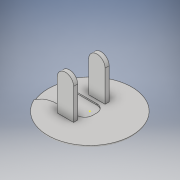
# Autodesk Inventor part: Replacemnet part(wall socket)
Saved by Autodesk Inventor 2018 (Build 220112000, 112)
## iProperties
Created: 2019-02-07
Part Number: Replacemnet part(wall socket)
Material: Generic
Document SubType Name: Modeling
Designer: This kid
Density: 1 g/cm^3
Appearance: Default
Author: This kid
Autodesk Inventor part; units mm, degrees
ref_plane "YZ Plane" through (0, 0, 0) normal (1, 0, 0) x (0, 1, 0)
ref_plane "XZ Plane" through (0, 0, 0) normal (0, 1, 0) x (-1, 0, 0)
ref_plane "XY Plane" through (0, 0, 0) normal (0, 0, 1) x (1, 0, 0)
sketch "Sketch1" plane through (0, 0, 0) normal (0, 1, 0) x (-1, 0, 0)
  circle A0 centre (0, 0) radius 16.9164
  dimension "d0" = 33.8328
  constraints: 1 centre point, 1 coincident
  measures "d0" diameter of A0
extrude "Extrusion1" add sketch "Sketch1" along normal blind 1
fillet "Fillet1" radius 1.016 1 edges at (16.9164, 0, 0)
sketch "Sketch2" plane through (0, 1, 0) normal (0, 1, 0) x (1, 0, 0)
  circle A0 centre (0, 0) radius 16.9164 projected
  line L0 (-0.1238, 7.1755) -> (0.6262, 7.1755) construction
  line L1 (-0.1238, 7.1755) -> (-0.8738, 7.1755) construction
  line L2 (0.6262, 7.1755) -> (-5.9778, 7.1755) construction
  line L3 (-5.9778, 7.1755) -> (-5.9778, 5.5245)
  line L4 (-5.9778, 5.5245) -> (0.6262, 5.5245)
  line L5 (0.6262, 5.5245) -> (0.6262, 7.1755)
  line L6 (0.6262, -7.1755) -> (-5.9778, -7.1755)
  line L7 (-5.9778, -7.1755) -> (-5.9778, -5.5245)
  line L8 (-5.9778, -5.5245) -> (0.6262, -5.5245)
  line L9 (0.6262, -5.5245) -> (0.6262, -7.1755)
  line L10 (0.6262, 6.35) -> (-5.9778, 6.35) construction
  line L11 (0.6262, -6.35) -> (-5.9778, -6.35) construction
  line L12 (-5.9778, 7.1755) -> (0.6262, 7.1755)
  line L13 (-2.6758, 6.35) -> (-2.6758, 16.7034) construction
  line L14 (-2.6758, -6.35) -> (-2.6758, -16.7034) construction
  line L15 (-5.9778, 7.1755) -> (-15.3192, 7.1755) construction
  line L16 (-5.9778, -7.1755) -> (-15.3192, -7.1755) construction
  line L17 (-15.3192, 7.1755) -> (-14.0913, 5.6461)
  line L18 (-12.4965, 4.5835) -> (-10.6485, 4.0497)
  line L19 (-10.6485, 4.0497) -> (-1.1572, 4.0497)
  line L20 (-10.6485, 4.0497) -> (-13.4621, 4.8624) construction
  line L21 (-13.4621, 4.8624) -> (-15.3192, 7.1755) construction
  line L22 (2.0178, 0.8747) -> (2.0178, 0)
  line L23 (2.0178, 0) -> (-20.8537, 0) construction
  line L24 (-15.3192, -7.1755) -> (-14.0913, -5.6461)
  line L25 (-12.4965, -4.5835) -> (-10.6485, -4.0497)
  line L26 (-10.6485, -4.0497) -> (-1.1572, -4.0497)
  line L27 (-10.6485, -4.0497) -> (-13.4621, -4.8624) construction
  line L28 (2.0178, -0.8747) -> (2.0178, 0)
  arc A1 (2.0178, 0.8747) -> (-1.1572, 4.0497) centre (-1.1572, 0.8747) ccw
  arc A2 (-1.1572, -4.0497) -> (2.0178, -0.8747) centre (-1.1572, -0.8747) ccw
  arc A3 (-14.0913, 5.6461) -> (-12.4965, 4.5835) centre (-11.6155, 7.6338) ccw
  arc A4 (-12.4965, -4.5835) -> (-14.0913, -5.6461) centre (-11.6155, -7.6338) ccw
  point P0 (-0.1238, -4.822)
  point P1 (-13.4621, 4.8624)
  point P2 (2.0178, 4.0497)
  point P3 (-13.4621, -4.8624)
  point P4 (2.0178, -4.0497)
  dimension "d17" = 6.604
  dimension "d18" = 1.651
  dimension "d20" = 12.7
  dimension "d21" = 6.604
  dimension "d22" = 1.651
  dimension "d28" = 3.175
  constraints: 58 end point, 12 point on circle, 9 point on line, 6 midpoint, 6 tangent, 4 centre point, 4 horizontal, 4 symmetric about line, 3 equal length, 3 equal radius, 2 perpendicular, 2 vertical, 1 collinear, 2 other
  measures "d17" distance of L4.end L3.end
  measures "d18" distance of L3.end L2.end
  measures "d20" distance between parallel lines of L11 L10
  measures "d21" distance of L9.end L6.end
  measures "d22" distance of L8.end L9.end
  measures "d28" radius of A1
sketch "Sketch3" plane through (0, 1, 0) normal (0, 1, 0) x (1, 0, 0)
  point P0 (0, 0)
extrude "Extrusion2" add sketch "Sketch2" along normal blind 15.9 contours L6 L7 L8 L9
extrude "Extrusion3" add sketch "Sketch2" along normal blind 15.9 contours L12 L5 L4 L3
fillet "Fillet2" radius 3.302 4 edges at (-5.9778, 16.9, 6.35) (0.6262, 16.9, 6.35) (-5.9778, 16.9, -6.35) (0.6262, 16.9, -6.35)
extrude "Extrusion4" cut sketch "Sketch2" against normal blind 0.5 contours L17 A3 L18 L19 A1 L22 L28 A2 L26 L25 A4 L24 A0 picked at (-4.321, -1.3499)
body "Solid1"
